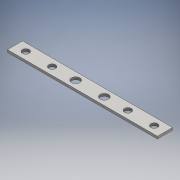
# Autodesk Inventor part: side2
Saved by Autodesk Inventor 2016 (Build 200138000, 138)
## iProperties
Created: 2016-09-24
Part Number: side2
Material: Generic
Document SubType Name: Modeling
Designer: Kevin G
Density: 1 g/cm^3
Appearance: Default
Author: Kevin G
Autodesk Inventor part; units mm, degrees
ref_plane "YZ Plane" through (0, 0, 0) normal (1, 0, 0) x (0, 1, 0)
ref_plane "XZ Plane" through (0, 0, 0) normal (0, 1, 0) x (-1, 0, 0)
ref_plane "XY Plane" through (0, 0, 0) normal (0, 0, 1) x (1, 0, 0)
sketch "Sketch1" plane through (0, 0, 0) normal (0, 0, 1) x (1, 0, 0)
  line L0 (-292.5876, 28.4768) -> (276.3724, 28.4768)
  line L1 (276.3724, 28.4768) -> (276.3724, -28.6732)
  line L2 (276.3724, -28.6732) -> (-292.5876, -28.6732)
  line L3 (-292.5876, -28.6732) -> (-292.5876, 28.4768)
  circle A0 centre (-251.9476, -0.0982) radius 13
  circle A1 centre (-151.8116, -0.0982) radius 13
  circle A2 centre (-62.4356, -0.0982) radius 16
  circle A3 centre (235.7324, -0.0982) radius 13
  circle A4 centre (135.5964, -0.0982) radius 13
  circle A5 centre (46.2204, -0.0982) radius 16
  point P0 (0, 0)
  point P1 (-193.5276, 9.4268)
  dimension "d0" = 26
  dimension "d1" = 26
  dimension "d2" = 32
  dimension "d3" = 26
  dimension "d4" = 26
  dimension "d5" = 32
  dimension "d6" = 568.96
  dimension "d7" = 57.15
  dimension "d8" = 40.64
  dimension "d9" = 140.776
  dimension "d10" = 230.152
  dimension "d11" = 230.152
  dimension "d12" = 40.64
  dimension "d13" = 140.776
  constraints: 8 end point, 6 centre point, 2 parallel, 1 horizontal, 1 perpendicular
  measures "d0" diameter of A0
  measures "d1" diameter of A1
  measures "d2" diameter of A2
  measures "d3" diameter of A3
  measures "d4" diameter of A4
  measures "d5" diameter of A5
  measures "d6" distance between parallel lines of L1 L3
  measures "d7" distance between parallel lines of L2 L0
  measures "d8" distance from line of A0.centre L3
  measures "d9" distance from line of A1.centre L3
  measures "d10" distance from line of A2.centre L3
  measures "d11" distance from line of A5.centre L1
  measures "d12" distance from line of A3.centre L1
  measures "d13" distance from line of A4.centre L1
extrude "Extrusion1" add sketch "Sketch1" along normal blind 9.525
body "Solid1"
